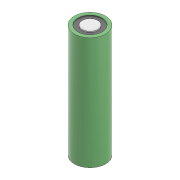
# Autodesk Inventor part: Batería
Saved by Autodesk Inventor 2022.3 (Build 263350000, 350)
## iProperties
Created: 2023-07-18
Part Number: Batería
Material: Genérico
Document SubType Name: Modeling
Designer: Usuario
Density: 1 g/cm^3
Appearance: Valor por defecto
Author: Usuario
Autodesk Inventor part; units mm, degrees
ref_plane "YZ Plane" through (0, 0, 0) normal (1, 0, 0) x (0, 1, 0)
ref_plane "XZ Plane" through (0, 0, 0) normal (0, 1, 0) x (-1, 0, 0)
ref_plane "XY Plane" through (0, 0, 0) normal (0, 0, 1) x (1, 0, 0)
sketch "Boceto1" plane through (0, 0, 0) normal (0, 1, 0) x (-1, 0, 0)
  circle A0 centre (0, 0) radius 9
  dimension "d0" = 18
  constraints: 1 centre point, 1 coincident
  measures "d0" diameter of A0
extrude "Extrusión1" add sketch "Boceto1" along normal blind 65
sketch "Boceto2" plane through (0, 65, 0) normal (0, 1, 0) x (1, 0, 0)
  circle A0 centre (0, 0) radius 4.5
  circle A1 centre (0, 0) radius 7
  dimension "d3" = 9
  dimension "d4" = 14
  constraints: 2 centre point, 2 coincident
  measures "d3" diameter of A0
  measures "d4" diameter of A1
extrude "Extrusión2" cut sketch "Boceto2" against normal blind 0.5
sketch "Boceto3" plane through (0, 0, 0) normal (0, -1, 0) x (1, 0, 0)
  circle A0 centre (0, 0) radius 7
  constraints: 1 centre point, 1 coincident
extrude "Extrusión3" cut sketch "Boceto3" against normal blind 0.1
